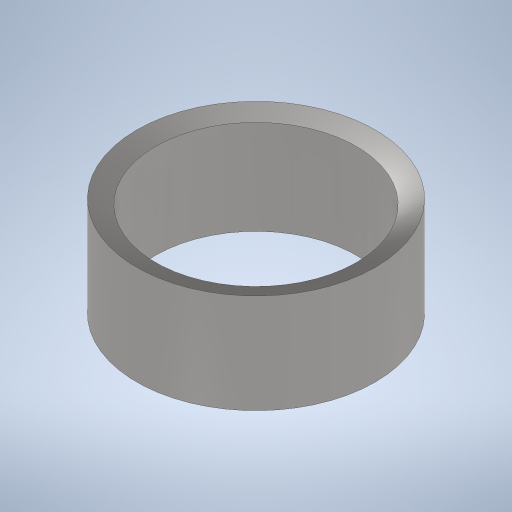
# Autodesk Inventor part: OringPressingRing
Saved by Autodesk Inventor 2024 (Build 280153000, 153)
## iProperties
Created: 2022-12-02
Part Number: OringPressingRing
Material: Stainless Steel, 440C
Document SubType Name: Modeling
Designer: kuzmin
Density: 7.75 g/cm^3
Appearance: Semi-Polished
Author: kuzmin
Autodesk Inventor part; units mm, degrees
ref_plane "YZ Plane" through (0, 0, 0) normal (1, 0, 0) x (0, 1, 0)
ref_plane "XZ Plane" through (0, 0, 0) normal (0, 1, 0) x (-1, 0, 0)
ref_plane "XY Plane" through (0, 0, 0) normal (0, 0, 1) x (1, 0, 0)
sketch "Sketch1" plane through (0, 0, 0) normal (0, 0, 1) x (1, 0, 0)
  line L0 (0, 0) -> (0, 15.2056) construction
  line L1 (20.4, 0) -> (20.4, 17)
  line L2 (20.4, 17) -> (17.2, 16.1426)
  line L3 (17.2, 16.1426) -> (17.2, 0)
  line L4 (17.2, 0) -> (20.4, 0)
  line L5 (17.2, 0) -> (20.4, 0)
  dimension "d0" = 40.8
  dimension "d1" = 75
  dimension "d2" = 17
  dimension "d5" = 34.4
  constraints: 12 end point, 2 vertical, 1 collinear, 1 horizontal alignment, 1 perpendicular
  measures "d0" diameter of L1 L0
  measures "d1" angle of L1 L2
  measures "d2" distance of L1.start L1.end
  measures "d5" diameter of L3 L0
revolve "Revolution1" add sketch "Sketch1" angle 360 about axis through (0, 0, 0) along (0, 1, 0)
body "Solid1"
